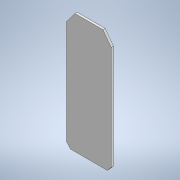
# Autodesk Inventor part: support_board_1
Saved by Autodesk Inventor 2020 (Build 240168000, 168)
## iProperties
Created: 2019-05-15
Part Number: support_board_1
Material: Generic
Document SubType Name: Modeling
Designer: psrob
Density: 1 g/cm^3
Appearance: Default
Author: psrob
Autodesk Inventor part; units mm, degrees
ref_plane "YZ Plane" through (0, 0, 0) normal (1, 0, 0) x (0, 1, 0)
ref_plane "XZ Plane" through (0, 0, 0) normal (0, 1, 0) x (-1, 0, 0)
ref_plane "XY Plane" through (0, 0, 0) normal (0, 0, 1) x (1, 0, 0)
sketch "Sketch1" plane through (0, 0, 0) normal (0, 0, 1) x (1, 0, 0)
  line L0 (25, -40) -> (28, -37) projected
  line L1 (28, -21.6) -> (28, -37) projected
  line L2 (39.9999, -8) -> (28, -21.6) projected
  line L3 (39.9999, 0) -> (39.9999, -8) projected
  line L4 (39.9999, 0) -> (20, 0) projected
  line L5 (20, 0) -> (20, -40) projected
  line L6 (25, -40) -> (20, -40) projected
  line L7 (15, -40) -> (12, -37) projected
  line L8 (15, -40) -> (20, -40) projected
  line L9 (20, 0) -> (20, -40) projected
  line L10 (0, 0) -> (20, 0) projected
  line L11 (0, 0) -> (0, -8) projected
  line L12 (0, -8) -> (12, -21.6) projected
  line L13 (12, -21.6) -> (12, -37) projected
  line L14 (40, 75.1166) -> (30, 85.1166) projected
  line L15 (40, 75.1166) -> (40, 85.1166) projected
  line L16 (25, 105.1166) -> (40, 85.1166) projected
  line L17 (25, 105.1166) -> (25, 115.1166) projected
  line L18 (25, 115.1166) -> (20, 115.1166) projected
  line L19 (20, 85.1166) -> (20, 115.1166) projected
  line L20 (30, 85.1166) -> (20, 85.1166) projected
  line L21 (0, 75.1166) -> (10, 85.1166) projected
  line L22 (10, 85.1166) -> (20, 85.1166) projected
  line L23 (20, 85.1166) -> (20, 115.1166) projected
  line L24 (15, 115.1166) -> (20, 115.1166) projected
  line L25 (15, 105.1166) -> (15, 115.1166) projected
  line L26 (15, 105.1166) -> (0, 85.1166) projected
  line L27 (0, 75.1166) -> (0, 85.1166) projected
  line L28 (20, 85.1166) -> (20, 95.1166)
  line L29 (20, 95.1166) -> (32.5, 95.1166)
  line L30 (20, 95.1166) -> (7.5, 95.1166)
  line L31 (20, 0) -> (20, -12)
  line L32 (20, -12) -> (36.4705, -12)
  line L33 (20, -12) -> (3.5294, -12)
  line L34 (0, 0) -> (0, 75.1166)
  line L35 (40, 75.1166) -> (39.9999, 0)
  dimension "d0" = 10
  dimension "d1" = 12
  constraints: 16 end point, 5 point on line, 2 midpoint, 1 perpendicular
  measures "d0" distance of L19.start L28.end
  measures "d1" distance of L4.end L31.end
extrude "Extrusion1" add sketch "Sketch1" along normal blind 2 contours L33 L12 L11 L10 L5 | L5 L4 L3 L2 L32 | L10 L34 L21 L22 L20 L14 L35 L4 | L14 L20 L19 L29 L16 L15 | L27 L26 L30 L19 L22 L21
body "Solid1"
